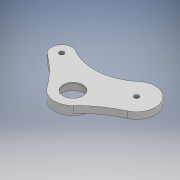
# Autodesk Inventor part: Arm 19X - parallel hinge
Saved by Autodesk Inventor 2017 (Build 210142000, 142)
## iProperties
Created: 2016-03-31
Part Number: Arm 19X - parallel hinge
Material: Generic
Document SubType Name: Modeling
Designer: alist
Density: 1 g/cm^3
Appearance: Default
Author: alist
## iProperties of the stored document Arm - parallel hinge_3DPrint.ipt
Created: 2017-01-15
Part Number: Arm - parallel hinge_3DPrint
Material: Generic
Document SubType Name: Modeling
Designer: Alistair
Density: 1 g/cm^3
Appearance: Default
Author: Alistair
Autodesk Inventor part; units mm, degrees
ref_plane "YZ Plane" through (0, 0, 0) normal (1, 0, 0) x (0, 1, 0)
ref_plane "XZ Plane" through (0, 0, 0) normal (0, 1, 0) x (-1, 0, 0)
ref_plane "XY Plane" through (0, 0, 0) normal (0, 0, 1) x (1, 0, 0)
sketch "Sketch1" plane through (0, 0, 0) normal (0, 0, 1) x (1, 0, 0)
  circle A0 centre (0, 0) radius 11
  circle A1 centre (-34.6, 24.3) radius 2.15
  circle A2 centre (34, 24) radius 2.15
  arc A3 (-29.8472, 32.3519) -> (-40.1494, 16.7749) centre (-34.6, 24.3) ccw
  arc A4 (41.1168, 8.5614) -> (22.9667, 36.9332) centre (34, 24) ccw
  arc A5 (-13.8132, -9.9093) -> (12.164, -11.8759) centre (0, 0) ccw
  arc A6 (-13.8132, -9.9093) -> (-40.1494, 16.7749) centre (-111.5168, -80) ccw
  arc A7 (41.1168, 8.5614) -> (12.164, -11.8759) centre (81.9412, -80) ccw
  arc A8 (-29.8472, 32.3519) -> (22.9667, 36.9332) centre (-6.6504, 71.6502) ccw
  line L0 (-111.5168, -80) -> (81.9412, -80) construction
  dimension "d0" = 22
  dimension "d1" = 4.3
  dimension "d2" = 4.3
  dimension "d4" = 34
  dimension "d5" = 34.6
  dimension "d6" = 7.2
  dimension "d8" = 6
  dimension "d9" = 80
  dimension "d16" = 24.3
  dimension "d17" = 24
  dimension "d20" = 17
  constraints: 12 point on circle, 9 centre point, 6 tangent, 2 coincident, 2 end point, 1 horizontal
  measures "d0" diameter of A0
  measures "d1" diameter of A1
  measures "d2" diameter of A2
  measures "d4" horizontal distance of A2.centre point (0, 0)
  measures "d5" horizontal distance of A1.centre point (0, 0)
  measures "d6" radial gap between concentric circles of A1 A3
  measures "d8" radial gap between concentric circles of A0 A5
  measures "d9" distance from line of L0 point (0, 0)
  measures "d16" vertical distance of point (0, 0) A1.centre
  measures "d17" vertical distance of point (0, 0) A2.centre
  measures "d20" radius of A4
extrude "Extrusion1" add sketch "Sketch1" along normal blind 6
sketch "Sketch2" plane through (0, 0, 6) normal (0, 0, 1) x (1, 0, 0)
  circle A0 centre (0, 0) radius 11 projected
  arc A1 (-13.8132, -9.9093) -> (12.164, -11.8759) centre (0, 0) ccw projected
  circle A2 centre (0, 0) radius 17
  circle A3 centre (0, 0) radius 11
  constraints: 2 coincident, 1 centre point, 1 concentric, 3 other
extrude "Extrusion2" add sketch "Sketch2" against normal blind 8
sketch "Sketch3" plane through (0, 0, 6) normal (0, 0, 1) x (1, 0, 0)
  circle A0 centre (0, 0) radius 11 projected
  circle A1 centre (0, 0) radius 9
  dimension "d21" = 18
  constraints: 1 centre point, 1 coincident
  measures "d21" diameter of A1
extrude "Extrusion3" add sketch "Sketch3" against normal blind 1
equation "\"d2\" = d1"
body "Solid1"
